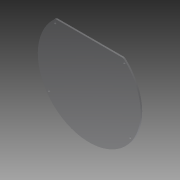
# Autodesk Inventor part: Top Plate
Saved by Autodesk Inventor 2015 (Build 190159000, 159)
## iProperties
Created: 2016-09-20
Part Number: Top Plate
Material: Generic
Document SubType Name: Modeling
Designer: James Yelland
Density: 1 g/cm^3
Appearance: Default
Author: James Yelland
Autodesk Inventor part; units mm, degrees
ref_plane "YZ Plane" through (0, 0, 0) normal (1, 0, 0) x (0, 1, 0)
ref_plane "XZ Plane" through (0, 0, 0) normal (0, 1, 0) x (-1, 0, 0)
ref_plane "XY Plane" through (0, 0, 0) normal (0, 0, 1) x (1, 0, 0)
sketch "Sketch1" plane through (0, 0, 0) normal (0, 1, 0) x (-1, 0, 0)
  circle A0 centre (-67.1751, 67.1751) radius 1.6
  circle A1 centre (67.1751, 67.1751) radius 1.6
  line L0 (0, 75) -> (64.2262, 75)
  line L1 (0, 75) -> (-64.2262, 75)
  arc A2 (-67.6065, 73.6842) -> (67.6065, 73.6842) centre (0, 0) ccw
  arc A3 (67.6065, 73.6842) -> (64.2262, 75) centre (64.2262, 70) ccw
  arc A4 (-64.2262, 75) -> (-67.6065, 73.6842) centre (-64.2262, 70) ccw
  circle A5 centre (-78.9896, -52.7792) radius 1.6
  circle A6 centre (78.9896, -52.7792) radius 1.6
  point P0 (66.1438, 75)
  point P1 (-66.1438, 75)
  dimension "d1" = 3.2
  dimension "d2" = 3.2
  dimension "d6" = 5
  dimension "d9" = 3.2
  dimension "d10" = 3.2
  constraints: 8 point on circle, 7 centre point, 4 end point, 4 tangent, 3 point on line, 1 coincident, 1 equal radius
  measures "d1" diameter of A0
  measures "d2" diameter of A1
  measures "d6" radius of A3
  measures "d9" diameter of A5
  measures "d10" diameter of A6
extrude "Extrusion1" add sketch "Sketch1" along normal blind 3
body "Solid1"
